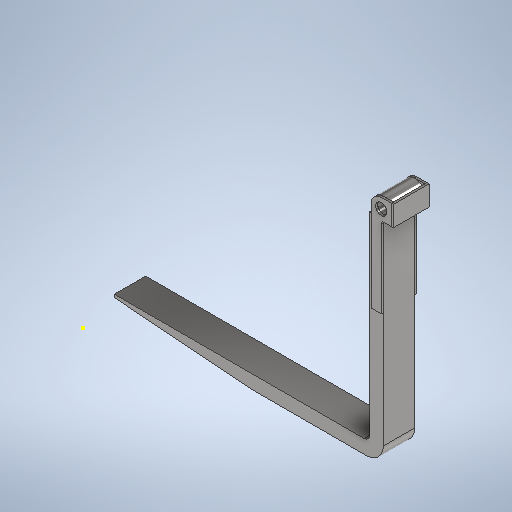
# Autodesk Inventor part: Arjun_Fork
Saved by Autodesk Inventor 2025 (Build 290162000, 162)
## iProperties
Created: 2024-10-18
Part Number: Arjun_Fork
Material: Generic
Document SubType Name: Modeling
Designer: pathl
Density: 1 g/cm^3
Appearance: Default
Author: pathl
Autodesk Inventor part; units mm, degrees
ref_plane "YZ Plane" through (0, 0, 0) normal (1, 0, 0) x (0, 1, 0)
ref_plane "XZ Plane" through (0, 0, 0) normal (0, 1, 0) x (-1, 0, 0)
sketch "Sketch1" plane through (0, 0, 0) normal (0, 0, 1) x (1, 0, 0)
  line L0 (610, 0) -> (1125, 0)
  line L1 (1200, 75) -> (1200, 950)
  arc A0 (1125, 0) -> (1200, 75) centre (1125, 75) ccw
  line L2 (0, 48.5) -> (0, 61)
  line L3 (0, 61) -> (1114, 61)
  line L4 (1139, 86) -> (1139, 950)
  line L5 (1139, 950) -> (1200, 950)
  arc A1 (1114, 61) -> (1139, 86) centre (1114, 86) ccw
  line L6 (0, 66.5) -> (0, 30.5)
  line L7 (0, 48.5) -> (610, 0)
  line L8 (1200, 950) -> (1200, 995)
  circle A2 centre (1200, 995) radius 45
  circle A3 centre (1200, 995) radius 25
  point P0 (0, 0)
  point P1 (1200, 0)
  dimension "d11" = 90
  dimension "d0" = 950
  dimension "d1" = 1200
  dimension "d2" = 75
  dimension "d3" = 61
  dimension "d4" = 61
  dimension "d5" = 25
  dimension "d8" = 12.5
  dimension "d9" = 610
  dimension "d10" = 50
  constraints: 18 end point, 4 point on circle, 4 point on line, 4 tangent, 3 centre point, 2 coincident, 1 horizontal, 1 midpoint, 1 perpendicular, 1 vertical alignment, 2 other
  measures "d0" distance of point (1200, 0) L1.end
  measures "d1" distance of point (0, 0) point (1200, 0)
  measures "d2" radius of A0
  measures "d3" distance between parallel lines of L1 L4
  measures "d4" distance between parallel lines of L0 L3
  measures "d5" radius of A1
  measures "d8" distance of L2.start L2.end
  measures "d9" horizontal distance of L0.start L2.start
  measures "d10" diameter of A3
extrude "Extrusion1" add sketch "Sketch1" along normal blind 140 contours L7 L2 L3 A1 L4 L5 L1 A0 L0
ref_plane "Work Plane1" through (0, 0, 70) normal (0, 0, 1) x (1, 0, 0)
sketch "Sketch2" plane through (0, 0, 70) normal (0, 0, 1) x (1, 0, 0)
  line L0 (1200, 75) -> (1200, 950) projected
  line L1 (1200, 950) -> (1200, 995)
  circle A0 centre (1200, 995) radius 45
  circle A1 centre (1200, 995) radius 25
  point P0 (0, 0)
  dimension "d14" = 90
  dimension "d13" = 50
  constraints: 2 coincident, 2 end point, 1 centre point, 1 vertical, 1 vertical alignment, 2 other
  measures "d13" diameter of A1
extrude "Extrusion2" add sketch "Sketch2" along normal mid plane 140
ref_plane "Work Plane2" through (0, 0, 70) normal (0, 0, 1) x (1, 0, 0)
sketch "Sketch3" plane through (0, 0, 70) normal (0, 0, 1) x (1, 0, 0)
  line L0 (1139, 950) -> (1139, 86) projected
  line L1 (1139, 950) -> (1164.8856, 966.8579)
  circle A0 centre (1200, 995) radius 45 projected
  line L2 (1139, 950) -> (1200, 950)
  line L3 (1200, 75) -> (1200, 950) projected
  arc A1 (1164.8856, 966.8579) -> (1200, 950) centre (1200, 995) ccw
  point P0 (0, 0)
  constraints: 4 end point, 3 point on circle, 1 centre point, 1 concentric, 1 perpendicular, 1 tangent
extrude "Extrusion3" add sketch "Sketch3" along normal mid plane 140 separate body contours L1 A0 L2
ref_plane "Work Plane3" through (0, 0, 280) normal (0, 0, 1) x (1, 0, 0)
sketch "Sketch4" plane through (0, 0, 280) normal (0, 0, 1) x (1, 0, 0)
  point P0 (0, 0)
ref_plane "Work Plane4" through (0, 0, 140) normal (0, 0, 1) x (1, 0, 0)
sketch "Sketch5" plane through (0, 0, 140) normal (0, 0, 1) x (1, 0, 0)
  circle A0 centre (1200, 995) radius 25 projected
  circle A1 centre (1200, 995) radius 25
  circle A2 centre (1200, 995) radius 45 projected
  line L0 (1155, 995) -> (1155, 590)
  line L1 (1155, 590) -> (1200, 590)
  line L2 (1200, 590) -> (1200, 937.5)
  line L3 (1155, 995) -> (1155, 590)
  line L4 (1155, 590) -> (1200, 590)
  line L5 (1200, 75) -> (1200, 950) projected
  line L6 (1200, 590) -> (1200, 950)
  line L7 (1212.5, 950) -> (1245, 950)
  line L8 (1245, 950) -> (1245, 1040)
  line L9 (1245, 1040) -> (1200, 1040)
  arc A3 (1200, 1040) -> (1155, 995) centre (1200, 995) ccw
  circle A4 centre (1200, 995) radius 25
  arc A5 (1212.5, 950) -> (1200, 937.5) centre (1212.5, 937.5) ccw
  point P0 (0, 0)
  dimension "d22" = 12.5
  dimension "d23" = 450
  constraints: 18 end point, 6 point on circle, 4 centre point, 4 tangent, 3 collinear, 3 point on line, 2 coincident, 2 concentric, 2 perpendicular, 1 vertical
  measures "d22" radius of A5
  measures "d23" distance of L1.end L9.end
extrude "Extrusion4" add sketch "Sketch5" along normal blind 9.5 separate body
ref_plane "Work Plane5" through (0, 0, 0) normal (0, 0, 1) x (1, 0, 0)
mirror "Mirror1" about plane through (0, 0, 0) normal (0, 0, 1) skipped copies 2
sketch "Sketch6" plane through (0, 0, 0) normal (0, 0, 1) x (1, 0, 0)
  circle A0 centre (1200, 995) radius 45 projected
  line L0 (1155, 995) -> (1155, 590)
  line L1 (1139, 950) -> (1139, 86) projected
  line L2 (1155, 590) -> (1200, 590)
  line L3 (1200, 75) -> (1200, 950) projected
  line L4 (1212.5, 950) -> (1245, 950) projected
  line L5 (1212.5, 950) -> (1245, 950)
  line L6 (1245, 1040) -> (1200, 1040) projected
  line L7 (1245, 950) -> (1245, 1040)
  line L8 (1245, 1040) -> (1200, 1040)
  arc A1 (1200, 1040) -> (1155, 995) centre (1200, 995) ccw
  circle A2 centre (1200, 995) radius 25
  line L9 (1200, 590) -> (1200, 937.5)
  arc A3 (1212.5, 950) -> (1200, 937.5) centre (1212.5, 937.5) ccw
  point P0 (0, 0)
  dimension "d27" = 12.5
  dimension "d28" = 450
  constraints: 12 end point, 5 point on circle, 4 tangent, 3 centre point, 3 point on line, 2 collinear, 2 perpendicular, 1 coincident, 1 horizontal, 1 parallel
  measures "d27" radius of A3
  measures "d28" distance of L2.end L6.end
extrude "Extrusion5" add sketch "Sketch6" against normal blind 9.5 separate body
sketch "Sketch7" plane through (1245, 950, 0) normal (1, 0, 0) x (0, 0, -1)
  line L0 (-140, 90) -> (-149.5, 90) projected
  line L1 (9.5, 90) -> (9.5, 0) projected
  line L2 (-149.5, 90) -> (9.5, 90)
  line L3 (9.5, 90) -> (9.5, 0)
  line L4 (9.5, 0) -> (-149.5, 0)
  line L5 (-149.5, 0) -> (-149.5, 90)
  point P0 (0, -950)
  constraints: 8 end point, 2 parallel, 1 horizontal, 1 perpendicular
extrude "Extrusion6" add sketch "Sketch7" along normal blind 9.5 separate body
ref_plane "Work Plane6" through (0, 0, 0) normal (0, 0, 1) x (1, 0, 0)
body "Solid1"
body "Solid2"
body "Solid3"
body "Solid4"
body "Solid5"
